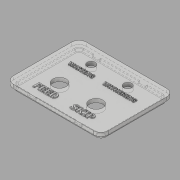
# Autodesk Inventor part: DispenserElectronicsBoxLidv2
Saved by Autodesk Inventor 2017 (Build 210142000, 142)
## iProperties
Created: 2017-05-31
Part Number: DispenserElectronicsBoxLidv2
Material: Generic
Document SubType Name: Modeling
Designer: gmarsh
Density: 1 g/cm^3
Appearance: Default
Author: gmarsh
Autodesk Inventor part; units mm, degrees
ref_plane "YZ Plane" through (0, 0, 0) normal (1, 0, 0) x (0, 1, 0)
ref_plane "XZ Plane" through (0, 0, 0) normal (0, 1, 0) x (-1, 0, 0)
ref_plane "XY Plane" through (0, 0, 0) normal (0, 0, 1) x (1, 0, 0)
sketch "Sketch1" plane through (0, 0, 0) normal (0, 0, 1) x (1, 0, 0)
  line L0 (-2, 58) -> (64, 58)
  line L1 (68, 54) -> (68, 6)
  line L2 (64, 2) -> (-2, 2)
  line L3 (-6, 6) -> (-6, 54)
  arc A0 (68, 54) -> (64, 58) centre (64, 54) ccw
  arc A1 (64, 2) -> (68, 6) centre (64, 6) ccw
  arc A2 (-6, 6) -> (-2, 2) centre (-2, 6) ccw
  arc A3 (-2, 58) -> (-6, 54) centre (-2, 54) ccw
  point P0 (0, 0)
  point P1 (31, 30)
  point P2 (31, 30)
  dimension "d0" = 4
  constraints: 8 end point, 8 point on circle, 8 tangent, 4 centre point, 3 equal radius, 2 parallel, 1 horizontal, 1 perpendicular
  measures "d0" radius of A0
extrude "Lid Surface Top" add sketch "Sketch1" along normal blind 3
thicken "Thicken1" operation add thickness 2 both sides no extend neighbours yes toward (-0.9972038, -0.0747301, 0) faces at (-5.9888, 5.7011, 2) (-6, 22, 1) (42, 2, 1) (66.7207, 3.0678, 2) (68, 38, 1) (66.2533, 57.305, 2) (20, 58, 1) (-4, 57.4641, 2)
sketch "Sketch2" plane through (0, 0, 0) normal (0, 0, -1) x (-1, 0, 0)
  line L0 (-63.5, 57.5) -> (1.5, 57.5)
  line L1 (5.5, 53.5) -> (5.5, 6.5)
  line L2 (1.5, 2.5) -> (-63.5, 2.5)
  line L3 (-67.5, 6.5) -> (-67.5, 53.5)
  arc A0 (5.5, 53.5) -> (1.5, 57.5) centre (1.5, 53.5) ccw
  arc A1 (1.5, 2.5) -> (5.5, 6.5) centre (1.5, 6.5) ccw
  arc A2 (-67.5, 6.5) -> (-63.5, 2.5) centre (-63.5, 6.5) ccw
  arc A3 (-63.5, 57.5) -> (-67.5, 53.5) centre (-63.5, 53.5) ccw
  point P0 (0, 0)
  point P1 (-62, 0)
  point P2 (-31, 30)
  point P3 (-31, 30)
  dimension "d5" = 4
  constraints: 8 end point, 8 point on circle, 8 tangent, 4 centre point, 3 equal radius, 2 parallel, 1 horizontal, 1 perpendicular
  measures "d5" radius of A0
surface extrude "Inside Lip" sketch "Sketch2" along normal blind 3 shown no curves L0 A0 L1 A1 L2 A2 L3 A3
thicken "Thicken2" operation add thickness 1 both sides no extend neighbours no toward (0, 1, 0) faces at (20.1667, 2.5, -1) (-4.2207, 3.5678, -2) (-5.5, 37.8333, -1) (-3.7533, 56.805, -2) (41.8333, 57.5, -1) (63.7989, 57.4888, -2) (67.5, 22.1667, -1) (63.7989, 2.5112, -1)
sketch "Sketch3" plane through (-1.5, 2.5, 0) normal (0, -1, 0) x (1, 0, 0)
  line L0 (14, -2) -> (10, -2)
  line L1 (10, 0) -> (14, 0)
  line L2 (65.5, 0) -> (1.5, 0) projected
  line L3 (52, 0) -> (48, 0)
  line L4 (48, -2) -> (52, -2)
  line L5 (1.5, 0) -> (65.5, 0) projected
  line L6 (9, 0) -> (15, 0)
  line L7 (15, 0) -> (15, -2)
  line L8 (15, -2) -> (9, -2)
  line L9 (9, -2) -> (9, 0)
  line L10 (47, 0) -> (53, 0)
  line L11 (53, 0) -> (53, -2)
  line L12 (53, -2) -> (47, -2)
  line L13 (47, -2) -> (47, 0)
  constraints: 24 end point, 6 parallel, 5 point on line, 4 horizontal, 2 perpendicular
extrude "Bottom Lip Notches" cut sketch "Sketch3" against normal blind 1
sketch "Sketch4" plane through (-1.5, 57.5, 0) normal (0, 1, 0) x (1, 0, 0)
  line L0 (47, 0) -> (51, 0)
  line L1 (51, 2) -> (47, 2)
  line L2 (9, 0) -> (13, 0)
  line L3 (52, 0) -> (46, 0)
  line L4 (46, 0) -> (46, 2)
  line L5 (46, 2) -> (52, 2)
  line L6 (52, 2) -> (52, 0)
  line L7 (8, 0) -> (14, 0)
  line L8 (14, 0) -> (14, 2)
  line L9 (8, 2) -> (8, 0)
  line L10 (14, 2) -> (8, 2)
  constraints: 22 end point, 5 horizontal, 4 parallel, 3 point on line, 2 perpendicular
extrude "Top Lip Notches" cut sketch "Sketch4" against normal blind 1
sketch "Sketch5" plane through (0, 0, 3) normal (0, 0, 1) x (1, 0, 0)
  circle A0 centre (16, 46) radius 3.25
  circle A1 centre (46, 46) radius 3.25
  circle A2 centre (16, 20) radius 5.5
  circle A3 centre (46, 20) radius 5.5
  point P0 (0, 0)
  point P1 (-17.6534, 30.861)
  dimension "d14" = 6.5
  dimension "d15" = 6.5
  dimension "d16" = 11
  dimension "d17" = 11
  constraints: 4 centre point
  measures "d14" diameter of A0
  measures "d15" diameter of A1
  measures "d16" diameter of A2
  measures "d17" diameter of A3
extrude "LED/Button Holes" cut sketch "Sketch5" against normal blind 3
sketch "Sketch6" plane through (64.4721, 51.1654, 3) normal (0, 0, 1) x (-1, 0, 0)
  line L0 (30.003, 11.9126) -> (13.6694, 11.9126) construction
  line L1 (13.6694, 11.9126) -> (13.6694, 17.9341) construction
  line L2 (13.6694, 17.9341) -> (30.003, 17.9341) construction
  line L3 (30.003, 17.9341) -> (30.003, 11.9126) construction
  line L4 (58.4416, 11.9127) -> (28.5678, 11.9127) construction
  line L5 (28.5678, 11.9127) -> (28.5678, 17.6268) construction
  line L6 (28.5678, 17.6268) -> (58.4416, 17.6268) construction
  line L7 (58.4416, 17.6268) -> (58.4416, 11.9127) construction
  line L8 (57.0144, 40.0169) -> (40.0373, 40.0169) construction
  line L9 (40.0373, 40.0169) -> (40.0373, 46.7475) construction
  line L10 (40.0373, 46.7475) -> (57.0144, 46.7475) construction
  line L11 (57.0144, 46.7475) -> (57.0144, 40.0169) construction
  line L12 (26.5675, 39.9675) -> (10.2936, 39.9675) construction
  line L13 (10.2936, 39.9675) -> (10.2936, 46.1958) construction
  line L14 (10.2936, 46.1958) -> (26.5675, 46.1958) construction
  line L15 (26.5675, 46.1958) -> (26.5675, 39.9675) construction
  line L16 (25.6846, 11.9729) -> (26.4684, 15.0729)
  line L17 (26.4684, 15.0729) -> (27.3225, 15.0729)
  line L18 (27.3225, 15.0729) -> (27.8199, 13.1561)
  line L19 (27.8199, 13.1561) -> (28.2998, 15.0729)
  line L20 (28.2998, 15.0729) -> (29.1564, 15.0729)
  line L21 (29.1564, 15.0729) -> (29.9402, 11.9729)
  line L22 (29.9402, 11.9729) -> (29.1313, 11.9729)
  line L23 (29.1313, 11.9729) -> (28.7042, 14.0479)
  line L24 (28.7042, 14.0479) -> (28.1867, 11.9729)
  line L25 (28.1867, 11.9729) -> (27.413, 11.9729)
  line L26 (27.413, 11.9729) -> (26.9206, 14.0504)
  line L27 (26.9206, 14.0504) -> (26.4734, 11.9729)
  line L28 (26.4734, 11.9729) -> (25.6846, 11.9729)
  line L29 (23.7578, 15.0729) -> (25.4259, 15.0729)
  line L30 (25.4259, 15.0729) -> (25.4259, 14.5328)
  line L31 (25.4259, 14.5328) -> (24.9812, 14.5328)
  line L32 (24.9812, 14.5328) -> (24.9812, 12.513)
  line L33 (24.9812, 12.513) -> (25.4259, 12.513)
  line L34 (25.4259, 12.513) -> (25.4259, 11.9729)
  line L35 (25.4259, 11.9729) -> (23.7578, 11.9729)
  line L36 (23.7578, 11.9729) -> (23.7578, 12.513)
  line L37 (23.7578, 12.513) -> (24.2024, 12.513)
  line L38 (24.2024, 12.513) -> (24.2024, 14.5328)
  line L39 (24.2024, 14.5328) -> (23.7578, 14.5328)
  line L40 (23.7578, 14.5328) -> (23.7578, 15.0729)
  line L41 (22.6449, 15.0729) -> (22.6449, 12.5632)
  line L42 (22.6449, 12.5632) -> (23.5618, 12.5632)
  line L43 (23.5618, 12.5632) -> (23.5618, 11.9729)
  line L44 (23.5618, 11.9729) -> (20.9492, 11.9729)
  line L45 (20.9492, 11.9729) -> (20.9492, 12.5632)
  line L46 (20.9492, 12.5632) -> (21.8661, 12.5632)
  line L47 (21.8661, 12.5632) -> (21.8661, 15.0729)
  line L48 (21.8661, 15.0729) -> (22.6449, 15.0729)
  line L49 (18.015, 15.0729) -> (18.7938, 15.0729)
  line L50 (18.7938, 15.0729) -> (18.7938, 13.6987)
  line L51 (18.7938, 13.6987) -> (19.8514, 13.6987)
  line L52 (19.8514, 13.6987) -> (19.8514, 15.0729)
  line L53 (19.8514, 15.0729) -> (20.6302, 15.0729)
  line L54 (20.6302, 15.0729) -> (20.6302, 11.9729)
  line L55 (20.6302, 11.9729) -> (19.8514, 11.9729)
  line L56 (19.8514, 11.9729) -> (19.8514, 13.1084)
  line L57 (19.8514, 13.1084) -> (18.7938, 13.1084)
  line L58 (18.7938, 13.1084) -> (18.7938, 11.9729)
  line L59 (18.7938, 11.9729) -> (18.015, 11.9729)
  line L60 (18.015, 11.9729) -> (18.015, 15.0729)
  line L61 (17.3719, 15.0729) -> (17.3719, 11.9729)
  line L62 (17.3719, 11.9729) -> (15.2768, 11.9729)
  line L63 (15.2768, 11.9729) -> (15.2768, 12.5632)
  line L64 (15.2768, 12.5632) -> (16.5981, 12.5632)
  line L65 (16.5981, 12.5632) -> (16.5981, 13.1084)
  line L66 (16.5981, 13.1084) -> (15.3798, 13.1084)
  line L67 (15.3798, 13.1084) -> (15.3798, 13.6987)
  line L68 (15.3798, 13.6987) -> (16.5981, 13.6987)
  line L69 (16.5981, 13.6987) -> (16.5981, 14.4825)
  line L70 (16.5981, 14.4825) -> (15.2768, 14.4825)
  line L71 (15.2768, 14.4825) -> (15.2768, 15.0729)
  line L72 (15.2768, 15.0729) -> (17.3719, 15.0729)
  line L73 (11.8853, 15.0729) -> (12.8324, 15.0729)
  line L74 (12.8324, 15.0729) -> (13.6941, 13.9349)
  line L75 (13.6941, 13.9349) -> (13.9755, 13.9349)
  line L76 (13.9755, 13.9349) -> (13.9755, 15.0729)
  line L77 (13.9755, 15.0729) -> (14.7492, 15.0729)
  line L78 (14.7492, 15.0729) -> (14.7492, 11.9729)
  line L79 (14.7492, 11.9729) -> (13.5032, 11.9729)
  spline S0 degree 2 poles (13.5032, 11.9729) (13.2444, 11.9729) (12.8626, 12.0382) (12.6993, 12.1387) knots 0 0 0 1 2 2 2
  spline S1 degree 2 poles (12.6993, 12.1387) (12.5335, 12.2442) (12.3375, 12.5733) (12.3375, 12.8245) knots 0 0 0 1 2 2 2
  spline S2 degree 2 poles (12.3375, 12.8245) (12.3375, 13.1787) (12.6591, 13.6234) (12.9279, 13.754) knots 0 0 0 1 2 2 2
  line L80 (12.9279, 13.754) -> (11.8853, 15.0729)
  spline S3 degree 2 poles (13.1364, 12.9225) (13.1364, 12.8044) (13.2268, 12.6361) (13.3298, 12.5909) knots 0 0 0 1 2 2 2
  spline S4 degree 2 poles (13.3298, 12.5909) (13.4027, 12.5607) (13.581, 12.5431) (13.7142, 12.5431) knots 0 0 0 1 2 2 2
  line L81 (13.7142, 12.5431) -> (13.9755, 12.5431)
  line L82 (13.9755, 12.5431) -> (13.9755, 13.3772)
  line L83 (13.9755, 13.3772) -> (13.7519, 13.3772)
  spline S5 degree 2 poles (13.7519, 13.3772) (13.5911, 13.3772) (13.3625, 13.337) (13.2846, 13.2742) knots 0 0 0 1 2 2 2
  spline S6 degree 2 poles (13.2846, 13.2742) (13.2093, 13.2139) (13.1364, 13.0531) (13.1364, 12.9225) knots 0 0 0 1 2 2 2
  line L84 (10.1118, 15.0729) -> (11.7798, 15.0729)
  line L85 (11.7798, 15.0729) -> (11.7798, 14.5328)
  line L86 (11.7798, 14.5328) -> (11.3352, 14.5328)
  line L87 (11.3352, 14.5328) -> (11.3352, 12.513)
  line L88 (11.3352, 12.513) -> (11.7798, 12.513)
  line L89 (11.7798, 12.513) -> (11.7798, 11.9729)
  line L90 (11.7798, 11.9729) -> (10.1118, 11.9729)
  line L91 (10.1118, 11.9729) -> (10.1118, 12.513)
  line L92 (10.1118, 12.513) -> (10.5564, 12.513)
  line L93 (10.5564, 12.513) -> (10.5564, 14.5328)
  line L94 (10.5564, 14.5328) -> (10.1118, 14.5328)
  line L95 (10.1118, 14.5328) -> (10.1118, 15.0729)
  line L96 (6.9389, 15.0729) -> (7.6875, 15.0729)
  line L97 (7.6875, 15.0729) -> (8.8833, 12.9124)
  line L98 (8.8833, 12.9124) -> (8.8833, 15.0729)
  line L99 (8.8833, 15.0729) -> (9.5943, 15.0729)
  line L100 (9.5943, 15.0729) -> (9.5943, 11.9729)
  line L101 (9.5943, 11.9729) -> (8.6396, 11.9729)
  line L102 (8.6396, 11.9729) -> (7.6498, 13.749)
  line L103 (7.6498, 13.749) -> (7.6498, 11.9729)
  line L104 (7.6498, 11.9729) -> (6.9389, 11.9729)
  line L105 (6.9389, 11.9729) -> (6.9389, 15.0729)
  spline S7 degree 2 poles (3.7208, 14.897) (3.9243, 14.9799) (4.575, 15.1382) (4.8915, 15.1382) knots 0 0 0 1 2 2 2
  spline S8 degree 2 poles (4.8915, 15.1382) (5.6225, 15.1382) (6.4892, 14.2941) (6.4892, 13.5204) knots 0 0 0 1 2 2 2
  spline S9 degree 2 poles (6.4892, 13.5204) (6.4892, 12.7918) (5.6225, 11.9126) (4.8689, 11.9126) knots 0 0 0 1 2 2 2
  spline S10 degree 2 poles (4.8689, 11.9126) (4.4795, 11.9126) (3.9922, 12.0608) (3.7334, 12.1864) knots 0 0 0 1 2 2 2
  line L106 (3.7334, 12.1864) -> (3.7334, 12.9149)
  line L107 (3.7334, 12.9149) -> (3.8037, 12.9149)
  spline S11 degree 2 poles (3.8037, 12.9149) (3.859, 12.8722) (4.07, 12.7089) (4.1705, 12.6537) knots 0 0 0 1 2 2 2
  spline S12 degree 2 poles (4.1705, 12.6537) (4.2861, 12.5858) (4.5926, 12.4904) (4.7634, 12.4904) knots 0 0 0 1 2 2 2
  spline S13 degree 2 poles (4.7634, 12.4904) (4.9618, 12.4904) (5.2909, 12.616) (5.4191, 12.7441) knots 0 0 0 1 2 2 2
  spline S14 degree 2 poles (5.4191, 12.7441) (5.5422, 12.8697) (5.6853, 13.2541) (5.6853, 13.5078) knots 0 0 0 1 2 2 2
  spline S15 degree 2 poles (5.6853, 13.5078) (5.6853, 14.0504) (5.1402, 14.5679) (4.6704, 14.5679) knots 0 0 0 1 2 2 2
  spline S16 degree 2 poles (4.6704, 14.5679) (4.6277, 14.5679) (4.5172, 14.5629) (4.4745, 14.5604) knots 0 0 0 1 2 2 2
  line L108 (4.4745, 14.5604) -> (4.4745, 13.9499)
  line L109 (4.4745, 13.9499) -> (5.0749, 13.9499)
  line L110 (5.0749, 13.9499) -> (5.0749, 13.3696)
  line L111 (5.0749, 13.3696) -> (3.7208, 13.3696)
  line L112 (3.7208, 13.3696) -> (3.7208, 14.897)
  line L113 (54.1232, 11.973) -> (54.907, 15.073)
  line L114 (54.907, 15.073) -> (55.7611, 15.073)
  line L115 (55.7611, 15.073) -> (56.2585, 13.1562)
  line L116 (56.2585, 13.1562) -> (56.7384, 15.073)
  line L117 (56.7384, 15.073) -> (57.595, 15.073)
  line L118 (57.595, 15.073) -> (58.3788, 11.973)
  line L119 (58.3788, 11.973) -> (57.5699, 11.973)
  line L120 (57.5699, 11.973) -> (57.1428, 14.0481)
  line L121 (57.1428, 14.0481) -> (56.6253, 11.973)
  line L122 (56.6253, 11.973) -> (55.8516, 11.973)
  line L123 (55.8516, 11.973) -> (55.3592, 14.0506)
  line L124 (55.3592, 14.0506) -> (54.912, 11.973)
  line L125 (54.912, 11.973) -> (54.1232, 11.973)
  line L126 (54.073, 15.073) -> (53.0254, 11.973)
  line L127 (53.0254, 11.973) -> (52.1763, 11.973)
  line L128 (52.1763, 11.973) -> (51.1287, 15.073)
  line L129 (51.1287, 15.073) -> (51.9301, 15.073)
  line L130 (51.9301, 15.073) -> (52.1235, 14.4399)
  line L131 (52.1235, 14.4399) -> (53.0983, 14.4399)
  line L132 (53.0983, 14.4399) -> (53.2942, 15.073)
  line L133 (53.2942, 15.073) -> (54.073, 15.073)
  line L134 (52.2944, 13.8772) -> (52.6109, 12.8523)
  line L135 (52.6109, 12.8523) -> (52.9299, 13.8772)
  line L136 (52.9299, 13.8772) -> (52.2944, 13.8772)
  line L137 (49.2773, 15.073) -> (50.9453, 15.073)
  line L138 (50.9453, 15.073) -> (50.9453, 14.5329)
  line L139 (50.9453, 14.5329) -> (50.5007, 14.5329)
  line L140 (50.5007, 14.5329) -> (50.5007, 12.5131)
  line L141 (50.5007, 12.5131) -> (50.9453, 12.5131)
  line L142 (50.9453, 12.5131) -> (50.9453, 11.973)
  line L143 (50.9453, 11.973) -> (49.2773, 11.973)
  line L144 (49.2773, 11.973) -> (49.2773, 12.5131)
  line L145 (49.2773, 12.5131) -> (49.7219, 12.5131)
  line L146 (49.7219, 12.5131) -> (49.7219, 14.5329)
  line L147 (49.7219, 14.5329) -> (49.2773, 14.5329)
  line L148 (49.2773, 14.5329) -> (49.2773, 15.073)
  line L149 (48.1644, 15.073) -> (48.1644, 12.5634)
  line L150 (48.1644, 12.5634) -> (49.0813, 12.5634)
  line L151 (49.0813, 12.5634) -> (49.0813, 11.973)
  line L152 (49.0813, 11.973) -> (46.4687, 11.973)
  line L153 (46.4687, 11.973) -> (46.4687, 12.5634)
  line L154 (46.4687, 12.5634) -> (47.3856, 12.5634)
  line L155 (47.3856, 12.5634) -> (47.3856, 15.073)
  line L156 (47.3856, 15.073) -> (48.1644, 15.073)
  line L157 (44.6072, 15.073) -> (46.2752, 15.073)
  line L158 (46.2752, 15.073) -> (46.2752, 14.5329)
  line L159 (46.2752, 14.5329) -> (45.8306, 14.5329)
  line L160 (45.8306, 14.5329) -> (45.8306, 12.5131)
  line L161 (45.8306, 12.5131) -> (46.2752, 12.5131)
  line L162 (46.2752, 12.5131) -> (46.2752, 11.973)
  line L163 (46.2752, 11.973) -> (44.6072, 11.973)
  line L164 (44.6072, 11.973) -> (44.6072, 12.5131)
  line L165 (44.6072, 12.5131) -> (45.0518, 12.5131)
  line L166 (45.0518, 12.5131) -> (45.0518, 14.5329)
  line L167 (45.0518, 14.5329) -> (44.6072, 14.5329)
  line L168 (44.6072, 14.5329) -> (44.6072, 15.073)
  line L169 (41.4343, 15.073) -> (42.1829, 15.073)
  line L170 (42.1829, 15.073) -> (43.3787, 12.9126)
  line L171 (43.3787, 12.9126) -> (43.3787, 15.073)
  line L172 (43.3787, 15.073) -> (44.0897, 15.073)
  line L173 (44.0897, 15.073) -> (44.0897, 11.973)
  line L174 (44.0897, 11.973) -> (43.135, 11.973)
  line L175 (43.135, 11.973) -> (42.1453, 13.7491)
  line L176 (42.1453, 13.7491) -> (42.1453, 11.973)
  line L177 (42.1453, 11.973) -> (41.4343, 11.973)
  line L178 (41.4343, 11.973) -> (41.4343, 15.073)
  spline S17 degree 2 poles (38.2162, 14.8972) (38.4197, 14.9801) (39.0704, 15.1383) (39.3869, 15.1383) knots 0 0 0 1 2 2 2
  spline S18 degree 2 poles (39.3869, 15.1383) (40.1179, 15.1383) (40.9846, 14.2942) (40.9846, 13.5205) knots 0 0 0 1 2 2 2
  spline S19 degree 2 poles (40.9846, 13.5205) (40.9846, 12.792) (40.1179, 11.9127) (39.3643, 11.9127) knots 0 0 0 1 2 2 2
  spline S20 degree 2 poles (39.3643, 11.9127) (38.9749, 11.9127) (38.4876, 12.0609) (38.2288, 12.1865) knots 0 0 0 1 2 2 2
  line L179 (38.2288, 12.1865) -> (38.2288, 12.9151)
  line L180 (38.2288, 12.9151) -> (38.2991, 12.9151)
  spline S21 degree 2 poles (38.2991, 12.9151) (38.3544, 12.8724) (38.5654, 12.7091) (38.6659, 12.6538) knots 0 0 0 1 2 2 2
  spline S22 degree 2 poles (38.6659, 12.6538) (38.7815, 12.586) (39.088, 12.4905) (39.2588, 12.4905) knots 0 0 0 1 2 2 2
  spline S23 degree 2 poles (39.2588, 12.4905) (39.4572, 12.4905) (39.7863, 12.6161) (39.9145, 12.7442) knots 0 0 0 1 2 2 2
  spline S24 degree 2 poles (39.9145, 12.7442) (40.0376, 12.8699) (40.1808, 13.2542) (40.1808, 13.5079) knots 0 0 0 1 2 2 2
  spline S25 degree 2 poles (40.1808, 13.5079) (40.1808, 14.0506) (39.6356, 14.5681) (39.1658, 14.5681) knots 0 0 0 1 2 2 2
  spline S26 degree 2 poles (39.1658, 14.5681) (39.1231, 14.5681) (39.0126, 14.563) (38.9699, 14.5605) knots 0 0 0 1 2 2 2
  line L181 (38.9699, 14.5605) -> (38.9699, 13.9501)
  line L182 (38.9699, 13.9501) -> (39.5703, 13.9501)
  line L183 (39.5703, 13.9501) -> (39.5703, 13.3698)
  line L184 (39.5703, 13.3698) -> (38.2162, 13.3698)
  line L185 (38.2162, 13.3698) -> (38.2162, 14.8972)
  line L186 (52.9943, 41.0072) -> (55.1771, 41.0072)
  line L187 (55.1771, 41.0072) -> (55.1771, 41.989)
  line L188 (55.1771, 41.989) -> (53.1671, 41.989)
  line L189 (53.1671, 41.989) -> (53.1671, 42.9793)
  line L190 (53.1671, 42.9793) -> (55.1771, 42.9793)
  line L191 (55.1771, 42.9793) -> (55.1771, 45.2169)
  line L192 (55.1771, 45.2169) -> (56.475, 45.2169)
  line L193 (56.475, 45.2169) -> (56.475, 40.0169)
  line L194 (56.475, 40.0169) -> (52.9943, 40.0169)
  line L195 (52.9943, 40.0169) -> (52.9943, 41.0072)
  line L196 (52.3201, 45.2169) -> (52.3201, 40.0169)
  line L197 (52.3201, 40.0169) -> (48.8056, 40.0169)
  line L198 (48.8056, 40.0169) -> (48.8056, 41.0072)
  line L199 (48.8056, 41.0072) -> (51.0222, 41.0072)
  line L200 (51.0222, 41.0072) -> (51.0222, 41.9216)
  line L201 (51.0222, 41.9216) -> (48.9784, 41.9216)
  line L202 (48.9784, 41.9216) -> (48.9784, 42.9119)
  line L203 (48.9784, 42.9119) -> (51.0222, 42.9119)
  line L204 (51.0222, 42.9119) -> (51.0222, 44.2267)
  line L205 (51.0222, 44.2267) -> (48.8056, 44.2267)
  line L206 (48.8056, 44.2267) -> (48.8056, 45.2169)
  line L207 (48.8056, 45.2169) -> (52.3201, 45.2169)
  line L208 (47.9207, 45.2169) -> (47.9207, 40.0169)
  line L209 (47.9207, 40.0169) -> (44.4063, 40.0169)
  line L210 (44.4063, 40.0169) -> (44.4063, 41.0072)
  line L211 (44.4063, 41.0072) -> (46.6228, 41.0072)
  line L212 (46.6228, 41.0072) -> (46.6228, 41.9216)
  line L213 (46.6228, 41.9216) -> (44.5791, 41.9216)
  line L214 (44.5791, 41.9216) -> (44.5791, 42.9119)
  line L215 (44.5791, 42.9119) -> (46.6228, 42.9119)
  line L216 (46.6228, 42.9119) -> (46.6228, 44.2267)
  line L217 (46.6228, 44.2267) -> (44.4063, 44.2267)
  line L218 (44.4063, 44.2267) -> (44.4063, 45.2169)
  line L219 (44.4063, 45.2169) -> (47.9207, 45.2169)
  spline S27 degree 2 poles (38.8818, 42.6211) (38.8818, 43.3502) (39.5181, 44.4963) (40.0027, 44.804) knots 0 0 0 1 2 2 2
  spline S28 degree 2 poles (40.0027, 44.804) (40.4073, 45.0652) (41.3596, 45.2169) (41.8948, 45.2169) knots 0 0 0 1 2 2 2
  line L220 (41.8948, 45.2169) -> (43.5214, 45.2169)
  line L221 (43.5214, 45.2169) -> (43.5214, 40.0169)
  line L222 (43.5214, 40.0169) -> (41.9116, 40.0169)
  spline S29 degree 2 poles (41.9116, 40.0169) (41.3638, 40.0169) (40.4073, 40.156) (39.9859, 40.4257) knots 0 0 0 1 2 2 2
  spline S30 degree 2 poles (39.9859, 40.4257) (39.476, 40.7544) (38.8818, 41.8668) (38.8818, 42.6211) knots 0 0 0 1 2 2 2
  spline S31 degree 2 poles (40.2219, 42.6127) (40.2219, 42.0986) (40.5758, 41.3654) (40.9382, 41.1589) knots 0 0 0 1 2 2 2
  spline S32 degree 2 poles (40.9382, 41.1589) (41.2037, 41.0156) (41.7852, 40.9861) (42.1898, 40.9861) knots 0 0 0 1 2 2 2
  line L223 (42.1898, 40.9861) -> (42.215, 40.9861)
  line L224 (42.215, 40.9861) -> (42.215, 44.2435)
  line L225 (42.215, 44.2435) -> (42.1898, 44.2435)
  spline S33 degree 2 poles (42.1898, 44.2435) (41.7515, 44.2435) (41.1489, 44.214) (40.875, 44.0412) knots 0 0 0 1 2 2 2
  spline S34 degree 2 poles (40.875, 44.0412) (40.5548, 43.839) (40.2219, 43.1268) (40.2219, 42.6127) knots 0 0 0 1 2 2 2
  spline S35 degree 2 poles (24.4226, 45.3529) (25.021, 45.3529) (25.9227, 45.1211) (26.3104, 44.9526) knots 0 0 0 1 2 2 2
  line L226 (26.3104, 44.9526) -> (26.3104, 43.7137)
  line L227 (26.3104, 43.7137) -> (26.1924, 43.7137)
  spline S36 degree 2 poles (26.1924, 43.7137) (25.8005, 44.0466) (24.8608, 44.4048) (24.4184, 44.4048) knots 0 0 0 1 2 2 2
  spline S37 degree 2 poles (24.4184, 44.4048) (24.3046, 44.4048) (23.938, 44.3542) (23.8284, 44.3036) knots 0 0 0 1 2 2 2
  spline S38 degree 2 poles (23.8284, 44.3036) (23.6936, 44.2446) (23.5039, 44.0297) (23.5039, 43.857) knots 0 0 0 1 2 2 2
  spline S39 degree 2 poles (23.5039, 43.857) (23.5039, 43.6589) (23.8116, 43.4145) (24.0223, 43.3597) knots 0 0 0 1 2 2 2
  spline S40 degree 2 poles (24.0223, 43.3597) (24.2877, 43.2881) (24.8903, 43.1659) (25.1558, 43.0732) knots 0 0 0 1 2 2 2
  spline S41 degree 2 poles (25.1558, 43.0732) (25.7584, 42.8625) (26.2809, 42.1419) (26.2809, 41.6025) knots 0 0 0 1 2 2 2
  spline S42 degree 2 poles (26.2809, 41.6025) (26.2809, 40.8735) (25.0463, 39.9675) (24.1192, 39.9675) knots 0 0 0 1 2 2 2
  spline S43 degree 2 poles (24.1192, 39.9675) (23.6557, 39.9675) (22.737, 40.1571) (22.3746, 40.3172) knots 0 0 0 1 2 2 2
  line L228 (22.3746, 40.3172) -> (22.3746, 41.5056)
  line L229 (22.3746, 41.5056) -> (22.4884, 41.5056)
  spline S44 degree 2 poles (22.4884, 41.5056) (22.7792, 41.257) (23.6135, 40.9156) (24.0518, 40.9156) knots 0 0 0 1 2 2 2
  spline S45 degree 2 poles (24.0518, 40.9156) (24.2245, 40.9156) (24.4942, 40.9662) (24.6459, 41.0336) knots 0 0 0 1 2 2 2
  spline S46 degree 2 poles (24.6459, 41.0336) (24.7681, 41.0884) (24.9451, 41.3075) (24.9451, 41.4424) knots 0 0 0 1 2 2 2
  spline S47 degree 2 poles (24.9451, 41.4424) (24.9451, 41.6446) (24.6628, 41.8764) (24.2582, 41.9691) knots 0 0 0 1 2 2 2
  spline S48 degree 2 poles (24.2582, 41.9691) (23.997, 42.0281) (23.5124, 42.1419) (23.2343, 42.2388) knots 0 0 0 1 2 2 2
  spline S49 degree 2 poles (23.2343, 42.2388) (22.6949, 42.4369) (22.1681, 43.0942) (22.1681, 43.6336) knots 0 0 0 1 2 2 2
  spline S50 degree 2 poles (22.1681, 43.6336) (22.1681, 44.409) (23.386, 45.3529) (24.4226, 45.3529) knots 0 0 0 1 2 2 2
  line L230 (16.9428, 45.2602) -> (18.5231, 45.2602)
  line L231 (18.5231, 45.2602) -> (19.9347, 43.149)
  line L232 (19.9347, 43.149) -> (20.1918, 43.503)
  line L233 (20.1918, 43.503) -> (20.1918, 45.2602)
  line L234 (20.1918, 45.2602) -> (21.4981, 45.2602)
  line L235 (21.4981, 45.2602) -> (21.4981, 40.0602)
  line L236 (21.4981, 40.0602) -> (20.1918, 40.0602)
  line L237 (20.1918, 40.0602) -> (20.1918, 42.3821)
  line L238 (20.1918, 42.3821) -> (18.5231, 40.0602)
  line L239 (18.5231, 40.0602) -> (17.0187, 40.0602)
  line L240 (17.0187, 40.0602) -> (18.8728, 42.4748)
  line L241 (18.8728, 42.4748) -> (16.9428, 45.2602)
  line L242 (13.9299, 45.2602) -> (16.7279, 45.2602)
  line L243 (16.7279, 45.2602) -> (16.7279, 44.3542)
  line L244 (16.7279, 44.3542) -> (15.9821, 44.3542)
  line L245 (15.9821, 44.3542) -> (15.9821, 40.9662)
  line L246 (15.9821, 40.9662) -> (16.7279, 40.9662)
  line L247 (16.7279, 40.9662) -> (16.7279, 40.0602)
  line L248 (16.7279, 40.0602) -> (13.9299, 40.0602)
  line L249 (13.9299, 40.0602) -> (13.9299, 40.9662)
  line L250 (13.9299, 40.9662) -> (14.6757, 40.9662)
  line L251 (14.6757, 40.9662) -> (14.6757, 44.3542)
  line L252 (14.6757, 44.3542) -> (13.9299, 44.3542)
  line L253 (13.9299, 44.3542) -> (13.9299, 45.2602)
  spline S51 degree 2 poles (9.0628, 41.6994) (9.0628, 42.0618) (9.2945, 42.7192) (9.5095, 42.9383) knots 0 0 0 1 2 2 2
  spline S52 degree 2 poles (9.5095, 42.9383) (9.6401, 43.0774) (9.9604, 43.3049) (10.15, 43.385) knots 0 0 0 1 2 2 2
  spline S53 degree 2 poles (10.15, 43.385) (10.3438, 43.4651) (10.7947, 43.5578) (11.0728, 43.5578) knots 0 0 0 1 2 2 2
  line L254 (11.0728, 43.5578) -> (11.7555, 43.5578)
  line L255 (11.7555, 43.5578) -> (11.7555, 45.2602)
  line L256 (11.7555, 45.2602) -> (13.0618, 45.2602)
  line L257 (13.0618, 45.2602) -> (13.0618, 40.0602)
  line L258 (13.0618, 40.0602) -> (11.0433, 40.0602)
  spline S54 degree 2 poles (11.0433, 40.0602) (10.5967, 40.0602) (9.9435, 40.2245) (9.678, 40.4015) knots 0 0 0 1 2 2 2
  spline S55 degree 2 poles (9.678, 40.4015) (9.383, 40.5996) (9.0628, 41.2485) (9.0628, 41.6994) knots 0 0 0 1 2 2 2
  spline S56 degree 2 poles (10.4028, 41.7331) (10.4028, 41.5098) (10.6135, 41.1937) (10.7568, 41.1348) knots 0 0 0 1 2 2 2
  spline S57 degree 2 poles (10.7568, 41.1348) (10.9422, 41.0547) (11.2793, 41.0294) (11.5701, 41.0294) knots 0 0 0 1 2 2 2
  line L259 (11.5701, 41.0294) -> (11.7555, 41.0294)
  line L260 (11.7555, 41.0294) -> (11.7555, 42.5886)
  line L261 (11.7555, 42.5886) -> (11.6628, 42.5886)
  spline S58 degree 2 poles (11.6628, 42.5886) (11.4816, 42.5886) (11.1529, 42.5801) (11.0307, 42.5591) knots 0 0 0 1 2 2 2
  spline S59 degree 2 poles (11.0307, 42.5591) (10.9253, 42.5422) (10.6936, 42.4411) (10.6304, 42.3779) knots 0 0 0 1 2 2 2
  spline S60 degree 2 poles (10.6304, 42.3779) (10.4955, 42.2514) (10.4028, 41.9691) (10.4028, 41.7331) knots 0 0 0 1 2 2 2
  point P0 (-17.6534, 30.861)
  constraints: 8 other
extrude "Text" add sketch "Sketch6" along normal blind 0.75
body "Solid1"
body "Srf1"
